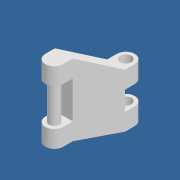
# Autodesk Inventor part: Crank1
Saved by Autodesk Inventor 2020 (Build 240168000, 168)
## iProperties
Created: 2019-12-22
Part Number: Crank1
Material: Generic
Document SubType Name: Modeling
Designer: Jack
Density: 1 g/cm^3
Appearance: Default
Author: Jack
Autodesk Inventor part; units mm, degrees
ref_plane "YZ Plane" through (0, 0, 0) normal (1, 0, 0) x (0, 1, 0)
ref_plane "XZ Plane" through (0, 0, 0) normal (0, 1, 0) x (-1, 0, 0)
ref_plane "XY Plane" through (0, 0, 0) normal (0, 0, 1) x (1, 0, 0)
sketch "Sketch2" plane through (0, 0, 0) normal (1, 0, 0) x (0, 1, 0)
  line L0 (0, 0) -> (32, 0)
  line L1 (0, 0) -> (-8, -23.4)
  line L2 (-8, -23.4) -> (16, -23.4)
  line L3 (16, -23.4) -> (32, 0)
  dimension "d4" = 32
  dimension "d32" = 24
  dimension "d34" = 8
  dimension "d35" = 23.4
  constraints: 8 end point, 2 horizontal
  measures "d4" distance of L0.start L0.end
  measures "d32" distance of L1.end L2.end
  measures "d34" horizontal distance of L0.start L1.end
  measures "d35" distance between parallel lines of L0 L2
extrude "Extrusion1" add sketch "Sketch2" along normal blind 8
sketch "Sketch7" plane through (0, -8, -23.4) normal (0, 0, -1) x (-1, 0, 0)
  line L0 (0, 24) -> (-8, 24) projected
  line L1 (-8, 24) -> (0, 24)
  line L2 (0, 24) -> (0, 16.3)
  line L3 (0, 16.3) -> (-8, 16.3)
  line L4 (-8, 16.3) -> (-8, 24)
  line L5 (0, 0) -> (-8, 0) projected
  line L6 (-8, 0) -> (0, 0)
  line L7 (0, 0) -> (0, 7.7)
  line L8 (0, 7.7) -> (-8, 7.7)
  line L9 (-8, 7.7) -> (-8, 0)
  point P0 (0, 8)
  dimension "d36" = 8
  dimension "d37" = 7.7
  dimension "d38" = 8
  dimension "d39" = 7.7
  constraints: 16 end point, 4 parallel, 2 horizontal, 2 perpendicular
  measures "d36" distance of L2.end L3.end
  measures "d37" distance of L1.end L2.end
  measures "d38" distance of L8.end L7.end
  measures "d39" distance of L7.end L6.end
extrude "Extrusion6" add sketch "Sketch7" along normal blind 8.3
sketch "Sketch8" plane through (0, 0, 0) normal (0, 0, 1) x (1, 0, 0)
  line L0 (0, 32) -> (8, 32) projected
  line L1 (8, 32) -> (0, 32)
  line L2 (0, 32) -> (0, 24.3)
  line L3 (0, 24.3) -> (8, 24.3)
  line L4 (8, 24.3) -> (8, 32)
  line L5 (8, 0) -> (0, 0)
  line L6 (0, 0) -> (0, 7.7)
  line L7 (0, 7.7) -> (8, 7.7)
  line L8 (8, 7.7) -> (8, 0)
  dimension "d42" = 8
  dimension "d43" = 7.7
  dimension "d44" = 8
  dimension "d45" = 7.7
  constraints: 16 end point, 4 parallel, 2 horizontal, 2 perpendicular, 1 point on line
  measures "d42" distance of L3.end L2.end
  measures "d43" distance of L2.end L1.end
  measures "d44" distance of L6.end L7.end
  measures "d45" distance of L5.end L6.end
extrude "Extrusion7" add sketch "Sketch8" along normal blind 8.3
sketch "Sketch9" plane through (0, 24.3, 0) normal (0, -1, 0) x (1, 0, 0)
  circle A0 centre (4, 4.3) radius 2.3
  line L0 (0, 0) -> (0, 8.3) projected
  line L1 (0, 8.3) -> (8, 8.3) projected
  dimension "d48" = 4.6
  dimension "d49" = 4
  dimension "d50" = 4
  constraints: 1 centre point
  measures "d48" diameter of A0
  measures "d49" distance from line of L0 A0.centre
  measures "d50" distance from line of L1 A0.centre
extrude "Extrusion8" add sketch "Sketch9" along normal up to surface (16.6 mm away)
sketch "Sketch10" plane through (0, 16, -23.4) normal (0, 1, 0) x (1, 0, 0)
  circle A0 centre (4, 4.3) radius 2.5
  line L0 (8, 0) -> (8, 8.3) projected
  line L1 (0, 8.3) -> (8, 8.3) projected
  point P0 (0, -23.4)
  dimension "d53" = 5
  dimension "d54" = 4
  dimension "d55" = 4
  constraints: 1 centre point
  measures "d53" diameter of A0
  measures "d54" distance from line of L0 A0.centre
  measures "d55" distance from line of L1 A0.centre
extrude "Extrusion9" cut sketch "Sketch10" against normal up to surface (24 mm away)
fillet "Fillet2" radius 4 8 edges at (0, 12.15, -31.7) (8, 12.15, -31.7) (8, -4.15, -31.7) (0, -4.15, -31.7) (0, 28.15, 8.3) (0, 3.85, 8.3) (8, 28.15, 8.3) (8, 3.85, 8.3)
body "Solid1"
